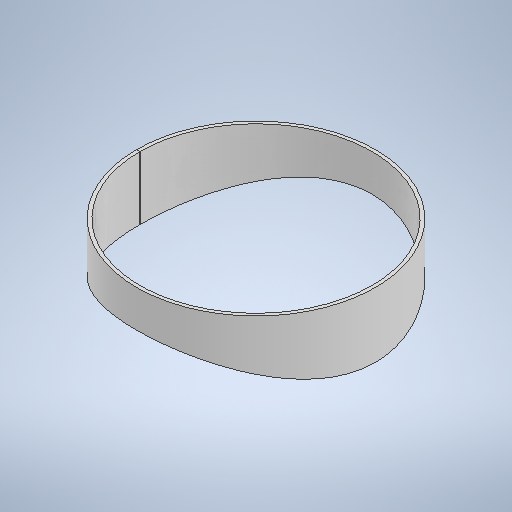
# Autodesk Inventor part: Ревиз. окно фильтра D1000
Saved by Autodesk Inventor 2025 (Build 290162010, 162A)
## iProperties
Created: 2025-02-12
Part Number: Ревиз. окно фильтра D1000
Material: Generic
Document SubType Name: Sheet Metal
Designer: pokla
Density: 1 g/cm^3
Appearance: Default
Flat Pattern Width: 11.579 cm
Flat Pattern Length: 131.684 cm
Flat Pattern Area: 1524.77 cm^2
Sheet Metal Rule: Default_mm
Sheet Metal Width: 115,790 mm
Sheet Metal Length: 1316,841 mm
Sheet Metal Area: 152476,805 mm^2
Author: pokla
Autodesk Inventor part; units mm, degrees
ref_plane "YZ Plane" through (0, 0, 0) normal (1, 0, 0) x (0, 1, 0)
ref_plane "XZ Plane" through (0, 0, 0) normal (0, 1, 0) x (-1, 0, 0)
ref_plane "XY Plane" through (0, 0, 0) normal (0, 0, 1) x (1, 0, 0)
sketch "Sketch1" plane through (0, 0, 0) normal (0, 1, 0) x (-1, 0, 0)
  line L0 (207, 66) -> (207, 0)
  line L1 (207, 0) -> (213, 0)
  line L2 (0, 0) -> (0, 109.131)
  line L3 (207, 66) -> (213, 66)
  line L4 (213, 0) -> (213, 66)
  line L5 (213, 0) -> (207, 0)
  line L6 (207, 0) -> (207, -100)
  line L7 (207, -100) -> (213, -100)
  line L8 (213, -100) -> (213, 0)
  point P0 (210, 0)
  dimension "d3" = 6
  dimension "d4" = 414
  dimension "d5" = 66
  dimension "d7" = 6
  dimension "d8" = 100
  constraints: 18 end point, 2 horizontal, 2 midpoint, 2 parallel, 2 perpendicular, 2 vertical, 1 horizontal alignment
  measures "d3" distance of L0.end L1.end
  measures "d4" diameter of L0 L2
  measures "d5" distance between parallel lines of L1 L3
  measures "d7" distance of L6.end L7.end
  measures "d8" distance of L7.end L5.start
revolve "Revolution1" add sketch "Sketch1" angle 359.9 about axis through (0, 0, 0) along (0, 0, 1)
sketch "Sketch2" plane through (0, 0, 0) normal (0, 1, 0) x (-1, 0, 0)
  circle A0 centre (0, -480.5) radius 480.5
  point P0 (0, 0)
  dimension "d9" = 961
  constraints: 2 vertical alignment, 2 other
extrude "Extrusion1" cut sketch "Sketch2" along normal through all both and the other way through all
equation "\"d4\" = Внутр_диам_ревиз_окна"
equation "\"d5\" = Длина_ревиз_окна"
equation "\"d7\" = d3"
equation "\"BendRadius\" = Thickness"
equation "\"BendReliefWidth\" = Thickness"
equation "\"BendReliefDepth\" = 0.5 * Thickness"
equation "\"CornerReliefSize\" = 4 * Thickness"
equation "\"MinimumRemnant\" = 2 * Thickness"
equation "\"TransitionRadius\" = BendRadius"
equation "\"JacobiRadiusSize\" = BendRadius"
equation "\"GapSize\" = Thickness"
equation "\"Внутр_диам_ревиз_окна\" = 414"
equation "\"Длина_ревиз_окна\" = 66"
equation "\"Thickness\" = 6"
body "Solid1"
